Autodesk Inventor part; units mm, degrees
(part 3 of 3)
sketch "Sketch4" plane through (0, 0, 0) normal (0, -1, 0) x (1, 0, 0)
  line L0 (-16.345, -5.1907) -> (6.6347, -5.1907) construction
  line L1 (6.6347, -5.1907) -> (6.6347, -8.929) construction
  line L2 (6.6347, -8.929) -> (-16.345, -8.929) construction
  line L3 (-16.345, -8.929) -> (-16.345, -5.1907) construction
  line L4 (-12.1827, 8.2163) -> (3.5843, 8.2163) construction
  line L5 (3.5843, 8.2163) -> (3.5843, 3.5647) construction
  line L6 (3.5843, 3.5647) -> (-12.1827, 3.5647) construction
  line L7 (-12.1827, 3.5647) -> (-12.1827, 8.2163) construction
  spline S0 degree 2 poles (-8.2562, 3.053) (-8.2439, 2.7183) (-7.9092, 2.4244) (-7.5011, 2.4244) knots 0 0 0 1 2 2 2
  spline S1 degree 2 poles (-7.5011, 2.4244) (-7.3623, 2.4244) (-6.9868, 2.5183) (-6.9133, 2.5551) knots 0 0 0 1 2 2 2
  line L8 (-6.9133, 2.5551) -> (-6.7868, 2.5551)
  line L9 (-6.7868, 2.5551) -> (-6.7868, 1.6734)
  spline S2 degree 2 poles (-6.7868, 1.6734) (-6.9745, 1.6285) (-7.4154, 1.5632) (-7.8684, 1.5632) knots 0 0 0 1 2 2 2
  spline S3 degree 2 poles (-7.8684, 1.5632) (-8.2684, 1.5632) (-8.8602, 1.7632) (-9.0602, 1.9428) knots 0 0 0 1 2 2 2
  spline S4 degree 2 poles (-9.0602, 1.9428) (-9.2521, 2.1224) (-9.448, 2.604) (-9.4643, 2.902) knots 0 0 0 1 2 2 2
  spline S5 degree 2 poles (-9.4643, 2.902) (-10.5827, 2.9673) (-11.8358, 4.3387) (-11.8358, 5.4897) knots 0 0 0 1 2 2 2
  spline S6 degree 2 poles (-11.8358, 5.4897) (-11.8358, 6.6979) (-10.4684, 8.0979) (-9.2602, 8.0979) knots 0 0 0 1 2 2 2
  spline S7 degree 2 poles (-9.2602, 8.0979) (-8.0602, 8.0979) (-6.6847, 6.6979) (-6.6847, 5.4897) knots 0 0 0 1 2 2 2
  spline S8 degree 2 poles (-6.6847, 5.4897) (-6.6847, 4.6) (-7.4888, 3.3102) (-8.2562, 3.053) knots 0 0 0 1 2 2 2
  spline S9 degree 2 poles (-8.3909, 4.2244) (-8.2031, 4.453) (-8.0235, 5.0775) (-8.0235, 5.4938) knots 0 0 0 1 2 2 2
  spline S10 degree 2 poles (-8.0235, 5.4938) (-8.0235, 5.9469) (-8.2317, 6.5755) (-8.399, 6.7714) knots 0 0 0 1 2 2 2
  spline S11 degree 2 poles (-8.399, 6.7714) (-8.5705, 6.9755) (-9.0154, 7.1551) (-9.2602, 7.1551) knots 0 0 0 1 2 2 2
  spline S12 degree 2 poles (-9.2602, 7.1551) (-9.5051, 7.1551) (-9.9378, 6.9795) (-10.1174, 6.7795) knots 0 0 0 1 2 2 2
  spline S13 degree 2 poles (-10.1174, 6.7795) (-10.2847, 6.5918) (-10.497, 5.9306) (-10.497, 5.4938) knots 0 0 0 1 2 2 2
  spline S14 degree 2 poles (-10.497, 5.4938) (-10.497, 5.0448) (-10.2929, 4.4163) (-10.1256, 4.2204) knots 0 0 0 1 2 2 2
  spline S15 degree 2 poles (-10.1256, 4.2204) (-9.9582, 4.0204) (-9.5051, 3.8326) (-9.2602, 3.8326) knots 0 0 0 1 2 2 2
  spline S16 degree 2 poles (-9.2602, 3.8326) (-9.0113, 3.8326) (-8.5623, 4.0244) (-8.3909, 4.2244) knots 0 0 0 1 2 2 2
  line L10 (-2.0113, 2.9918) -> (-3.2235, 2.9918)
  line L11 (-3.2235, 2.9918) -> (-3.2235, 3.4081)
  spline S17 degree 2 poles (-3.2235, 3.4081) (-3.5582, 3.151) (-4.1174, 2.8857) (-4.5011, 2.8857) knots 0 0 0 1 2 2 2
  spline S18 degree 2 poles (-4.5011, 2.8857) (-5.1256, 2.8857) (-5.799, 3.604) (-5.799, 4.3061) knots 0 0 0 1 2 2 2
  line L12 (-5.799, 4.3061) -> (-5.799, 6.7632)
  line L13 (-5.799, 6.7632) -> (-4.5868, 6.7632)
  line L14 (-4.5868, 6.7632) -> (-4.5868, 4.8897)
  spline S19 degree 2 poles (-4.5868, 4.8897) (-4.5868, 4.604) (-4.55, 4.2244) (-4.4807, 4.102) knots 0 0 0 1 2 2 2
  spline S20 degree 2 poles (-4.4807, 4.102) (-4.4194, 3.9755) (-4.1623, 3.8612) (-3.9296, 3.8612) knots 0 0 0 1 2 2 2
  spline S21 degree 2 poles (-3.9296, 3.8612) (-3.7745, 3.8612) (-3.399, 3.9755) (-3.2235, 4.0857) knots 0 0 0 1 2 2 2
  line L15 (-3.2235, 4.0857) -> (-3.2235, 6.7632)
  line L16 (-3.2235, 6.7632) -> (-2.0113, 6.7632)
  line L17 (-2.0113, 6.7632) -> (-2.0113, 2.9918)
  line L18 (0.3438, 2.9918) -> (-0.8684, 2.9918)
  line L19 (-0.8684, 2.9918) -> (-0.8684, 6.7632)
  line L20 (-0.8684, 6.7632) -> (0.3438, 6.7632)
  line L21 (0.3438, 6.7632) -> (0.3438, 2.9918)
  line L22 (0.3765, 7.2979) -> (-0.9011, 7.2979)
  line L23 (-0.9011, 7.2979) -> (-0.9011, 8.2163)
  line L24 (-0.9011, 8.2163) -> (0.3765, 8.2163)
  line L25 (0.3765, 8.2163) -> (0.3765, 7.2979)
  spline S22 degree 2 poles (3.4459, 2.8897) (2.952, 2.8897) (2.1357, 3.1265) (1.8336, 3.3714) knots 0 0 0 1 2 2 2
  spline S23 degree 2 poles (1.8336, 3.3714) (1.5357, 3.6163) (1.2051, 4.3591) (1.2051, 4.8612) knots 0 0 0 1 2 2 2
  spline S24 degree 2 poles (1.2051, 4.8612) (1.2051, 5.3877) (1.5561, 6.1551) (1.8744, 6.404) knots 0 0 0 1 2 2 2
  spline S25 degree 2 poles (1.8744, 6.404) (2.1806, 6.6448) (2.9765, 6.8653) (3.4091, 6.8653) knots 0 0 0 1 2 2 2
  spline S26 degree 2 poles (3.4091, 6.8653) (3.7928, 6.8653) (4.4459, 6.6979) (4.7275, 6.5632) knots 0 0 0 1 2 2 2
  line L26 (4.7275, 6.5632) -> (4.7275, 5.5306)
  line L27 (4.7275, 5.5306) -> (4.5561, 5.5306)
  spline S27 degree 2 poles (4.5561, 5.5306) (4.4867, 5.5918) (4.2867, 5.7551) (4.1438, 5.8326) knots 0 0 0 1 2 2 2
  spline S28 degree 2 poles (4.1438, 5.8326) (4.0051, 5.9061) (3.6785, 6.004) (3.4622, 6.004) knots 0 0 0 1 2 2 2
  spline S29 degree 2 poles (3.4622, 6.004) (2.9765, 6.004) (2.4581, 5.3877) (2.4581, 4.8612) knots 0 0 0 1 2 2 2
  spline S30 degree 2 poles (2.4581, 4.8612) (2.4581, 4.3142) (2.9928, 3.751) (3.4785, 3.751) knots 0 0 0 1 2 2 2
  spline S31 degree 2 poles (3.4785, 3.751) (3.7071, 3.751) (4.0744, 3.8571) (4.1928, 3.9265) knots 0 0 0 1 2 2 2
  spline S32 degree 2 poles (4.1928, 3.9265) (4.3071, 3.9918) (4.4826, 4.1428) (4.5561, 4.2122) knots 0 0 0 1 2 2 2
  line L28 (4.5561, 4.2122) -> (4.7275, 4.2122)
  line L29 (4.7275, 4.2122) -> (4.7275, 3.1836)
  spline S33 degree 2 poles (4.7275, 3.1836) (4.4418, 3.0489) (3.8214, 2.8897) (3.4459, 2.8897) knots 0 0 0 1 2 2 2
  line L30 (9.5275, 2.9918) -> (8.1234, 2.9918)
  line L31 (8.1234, 2.9918) -> (7.0663, 4.6326)
  line L32 (7.0663, 4.6326) -> (6.7398, 4.2285)
  line L33 (6.7398, 4.2285) -> (6.7398, 2.9918)
  line L34 (6.7398, 2.9918) -> (5.5275, 2.9918)
  line L35 (5.5275, 2.9918) -> (5.5275, 8.2163)
  line L36 (5.5275, 8.2163) -> (6.7398, 8.2163)
  line L37 (6.7398, 8.2163) -> (6.7398, 5.1061)
  line L38 (6.7398, 5.1061) -> (8.0336, 6.7632)
  line L39 (8.0336, 6.7632) -> (9.4295, 6.7632)
  line L40 (9.4295, 6.7632) -> (8.0785, 5.1387)
  line L41 (8.0785, 5.1387) -> (9.5275, 2.9918)
  line L42 (12.8744, 5.6122) -> (12.7683, 5.6122)
  spline S34 degree 2 poles (12.7683, 5.6122) (12.6908, 5.6408) (12.3479, 5.6653) (12.2336, 5.6653) knots 0 0 0 1 2 2 2
  spline S35 degree 2 poles (12.2336, 5.6653) (11.9765, 5.6653) (11.5806, 5.6) (11.352, 5.5183) knots 0 0 0 1 2 2 2
  line L43 (11.352, 5.5183) -> (11.352, 2.9918)
  line L44 (11.352, 2.9918) -> (10.1398, 2.9918)
  line L45 (10.1398, 2.9918) -> (10.1398, 6.7632)
  line L46 (10.1398, 6.7632) -> (11.352, 6.7632)
  line L47 (11.352, 6.7632) -> (11.352, 6.2081)
  spline S36 degree 2 poles (11.352, 6.2081) (11.752, 6.551) (12.3398, 6.7755) (12.5887, 6.7755) knots 0 0 0 1 2 2 2
  spline S37 degree 2 poles (12.5887, 6.7755) (12.654, 6.7755) (12.8132, 6.7673) (12.8744, 6.7632) knots 0 0 0 1 2 2 2
  line L48 (12.8744, 6.7632) -> (12.8744, 5.6122)
  line L49 (-13.0732, -8.3254) -> (-14.0161, -8.3254)
  line L50 (-14.0161, -8.3254) -> (-14.834, -7.2258)
  line L51 (-14.834, -7.2258) -> (-15.194, -7.2258)
  line L52 (-15.194, -7.2258) -> (-15.194, -8.3254)
  line L53 (-15.194, -8.3254) -> (-15.963, -8.3254)
  line L54 (-15.963, -8.3254) -> (-15.963, -5.3254)
  line L55 (-15.963, -5.3254) -> (-14.665, -5.3254)
  spline S38 degree 2 poles (-14.665, -5.3254) (-14.3981, -5.3254) (-14.0161, -5.3866) (-13.8495, -5.4871) knots 0 0 0 1 2 2 2
  spline S39 degree 2 poles (-13.8495, -5.4871) (-13.6781, -5.5875) (-13.4797, -5.9083) (-13.4797, -6.1507) knots 0 0 0 1 2 2 2
  spline S40 degree 2 poles (-13.4797, -6.1507) (-13.4797, -6.4813) (-13.7883, -6.9026) (-14.0748, -7.0397) knots 0 0 0 1 2 2 2
  line L56 (-14.0748, -7.0397) -> (-13.0732, -8.3254)
  spline S41 degree 2 poles (-14.2805, -6.2438) (-14.2805, -6.1311) (-14.3736, -5.9695) (-14.4863, -5.923) knots 0 0 0 1 2 2 2
  spline S42 degree 2 poles (-14.4863, -5.923) (-14.5646, -5.8911) (-14.7752, -5.8764) (-14.9148, -5.8764) knots 0 0 0 1 2 2 2
  line L57 (-14.9148, -5.8764) -> (-15.194, -5.8764)
  line L58 (-15.194, -5.8764) -> (-15.194, -6.6846)
  line L59 (-15.194, -6.6846) -> (-14.9565, -6.6846)
  spline S43 degree 2 poles (-14.9565, -6.6846) (-14.7703, -6.6846) (-14.5205, -6.6479) (-14.4348, -6.5842) knots 0 0 0 1 2 2 2
  spline S44 degree 2 poles (-14.4348, -6.5842) (-14.354, -6.5205) (-14.2805, -6.3711) (-14.2805, -6.2438) knots 0 0 0 1 2 2 2
  spline S45 degree 2 poles (-10.4601, -7.194) (-10.4601, -7.7524) (-11.1116, -8.3964) (-11.6993, -8.3964) knots 0 0 0 1 2 2 2
  spline S46 degree 2 poles (-11.6993, -8.3964) (-12.2895, -8.3964) (-12.941, -7.7524) (-12.941, -7.194) knots 0 0 0 1 2 2 2
  spline S47 degree 2 poles (-12.941, -7.194) (-12.941, -6.6332) (-12.2846, -5.9915) (-11.6993, -5.9915) knots 0 0 0 1 2 2 2
  spline S48 degree 2 poles (-11.6993, -5.9915) (-11.1067, -5.9915) (-10.4601, -6.6356) (-10.4601, -7.194) knots 0 0 0 1 2 2 2
  spline S49 degree 2 poles (-11.354, -7.745) (-11.283, -7.6569) (-11.212, -7.4144) (-11.212, -7.1989) knots 0 0 0 1 2 2 2
  spline S50 degree 2 poles (-11.212, -7.1989) (-11.212, -7.0005) (-11.2854, -6.7311) (-11.3491, -6.6503) knots 0 0 0 1 2 2 2
  spline S51 degree 2 poles (-11.3491, -6.6503) (-11.4128, -6.5671) (-11.5965, -6.4985) (-11.6993, -6.4985) knots 0 0 0 1 2 2 2
  spline S52 degree 2 poles (-11.6993, -6.4985) (-11.8046, -6.4985) (-11.9687, -6.5548) (-12.0446, -6.6405) knots 0 0 0 1 2 2 2
  spline S53 degree 2 poles (-12.0446, -6.6405) (-12.1108, -6.7189) (-12.1891, -6.9907) (-12.1891, -7.1989) knots 0 0 0 1 2 2 2
  spline S54 degree 2 poles (-12.1891, -7.1989) (-12.1891, -7.385) (-12.1205, -7.6569) (-12.0544, -7.7377) knots 0 0 0 1 2 2 2
  spline S55 degree 2 poles (-12.0544, -7.7377) (-11.9883, -7.816) (-11.8095, -7.8895) (-11.6944, -7.8895) knots 0 0 0 1 2 2 2
  spline S56 degree 2 poles (-11.6944, -7.8895) (-11.5965, -7.8895) (-11.4152, -7.8234) (-11.354, -7.745) knots 0 0 0 1 2 2 2
  spline S57 degree 2 poles (-7.5801, -7.1622) (-7.5801, -7.696) (-8.1703, -8.3695) (-8.6112, -8.3695) knots 0 0 0 1 2 2 2
  spline S58 degree 2 poles (-8.6112, -8.3695) (-8.7997, -8.3695) (-9.0838, -8.2887) (-9.2136, -8.2128) knots 0 0 0 1 2 2 2
  line L60 (-9.2136, -8.2128) -> (-9.243, -8.3254)
  line L61 (-9.243, -8.3254) -> (-9.941, -8.3254)
  line L62 (-9.941, -8.3254) -> (-9.941, -5.1907)
  line L63 (-9.941, -5.1907) -> (-9.2136, -5.1907)
  line L64 (-9.2136, -5.1907) -> (-9.2136, -6.3001)
  spline S59 degree 2 poles (-9.2136, -6.3001) (-9.0471, -6.1654) (-8.6993, -6.0013) (-8.4716, -6.0013) knots 0 0 0 1 2 2 2
  spline S60 degree 2 poles (-8.4716, -6.0013) (-8.043, -6.0013) (-7.5801, -6.6185) (-7.5801, -7.1622) knots 0 0 0 1 2 2 2
  spline S61 degree 2 poles (-8.3271, -7.1793) (-8.3271, -6.8781) (-8.5328, -6.5524) (-8.7948, -6.5524) knots 0 0 0 1 2 2 2
  spline S62 degree 2 poles (-8.7948, -6.5524) (-8.8977, -6.5524) (-9.1157, -6.6136) (-9.2136, -6.6724) knots 0 0 0 1 2 2 2
  line L65 (-9.2136, -6.6724) -> (-9.2136, -7.8038)
  spline S63 degree 2 poles (-9.2136, -7.8038) (-9.1352, -7.8332) (-8.9957, -7.8528) (-8.8952, -7.8528) knots 0 0 0 1 2 2 2
  spline S64 degree 2 poles (-8.8952, -7.8528) (-8.6087, -7.8528) (-8.3271, -7.5148) (-8.3271, -7.1793) knots 0 0 0 1 2 2 2
  spline S65 degree 2 poles (-4.7418, -7.194) (-4.7418, -7.7524) (-5.3932, -8.3964) (-5.981, -8.3964) knots 0 0 0 1 2 2 2
  spline S66 degree 2 poles (-5.981, -8.3964) (-6.5712, -8.3964) (-7.2226, -7.7524) (-7.2226, -7.194) knots 0 0 0 1 2 2 2
  spline S67 degree 2 poles (-7.2226, -7.194) (-7.2226, -6.6332) (-6.5663, -5.9915) (-5.981, -5.9915) knots 0 0 0 1 2 2 2
  spline S68 degree 2 poles (-5.981, -5.9915) (-5.3883, -5.9915) (-4.7418, -6.6356) (-4.7418, -7.194) knots 0 0 0 1 2 2 2
  spline S69 degree 2 poles (-5.6357, -7.745) (-5.5646, -7.6569) (-5.4936, -7.4144) (-5.4936, -7.1989) knots 0 0 0 1 2 2 2
  spline S70 degree 2 poles (-5.4936, -7.1989) (-5.4936, -7.0005) (-5.5671, -6.7311) (-5.6308, -6.6503) knots 0 0 0 1 2 2 2
  spline S71 degree 2 poles (-5.6308, -6.6503) (-5.6944, -6.5671) (-5.8781, -6.4985) (-5.981, -6.4985) knots 0 0 0 1 2 2 2
  spline S72 degree 2 poles (-5.981, -6.4985) (-6.0863, -6.4985) (-6.2503, -6.5548) (-6.3263, -6.6405) knots 0 0 0 1 2 2 2
  spline S73 degree 2 poles (-6.3263, -6.6405) (-6.3924, -6.7189) (-6.4708, -6.9907) (-6.4708, -7.1989) knots 0 0 0 1 2 2 2
  spline S74 degree 2 poles (-6.4708, -7.1989) (-6.4708, -7.385) (-6.4022, -7.6569) (-6.3361, -7.7377) knots 0 0 0 1 2 2 2
  spline S75 degree 2 poles (-6.3361, -7.7377) (-6.2699, -7.816) (-6.0912, -7.8895) (-5.9761, -7.8895) knots 0 0 0 1 2 2 2
  spline S76 degree 2 poles (-5.9761, -7.8895) (-5.8781, -7.8895) (-5.6969, -7.8234) (-5.6357, -7.745) knots 0 0 0 1 2 2 2
  spline S77 degree 2 poles (-1.6144, -7.4071) (-1.6144, -7.625) (-1.7908, -7.9679) (-1.9426, -8.0805) knots 0 0 0 1 2 2 2
  spline S78 degree 2 poles (-1.9426, -8.0805) (-2.1214, -8.2128) (-2.545, -8.3254) (-2.8732, -8.3254) knots 0 0 0 1 2 2 2
  line L66 (-2.8732, -8.3254) -> (-4.1834, -8.3254)
  line L67 (-4.1834, -8.3254) -> (-4.1834, -5.3254)
  line L68 (-4.1834, -5.3254) -> (-3.0177, -5.3254)
  spline S79 degree 2 poles (-3.0177, -5.3254) (-2.6552, -5.3254) (-2.3197, -5.3744) (-2.1532, -5.4552) knots 0 0 0 1 2 2 2
  spline S80 degree 2 poles (-2.1532, -5.4552) (-1.9818, -5.5434) (-1.8152, -5.8348) (-1.8152, -6.0234) knots 0 0 0 1 2 2 2
  spline S81 degree 2 poles (-1.8152, -6.0234) (-1.8152, -6.2413) (-2.0454, -6.572) (-2.2561, -6.665) knots 0 0 0 1 2 2 2
  line L69 (-2.2561, -6.665) -> (-2.2561, -6.6822)
  spline S82 degree 2 poles (-2.2561, -6.6822) (-1.9597, -6.7409) (-1.6144, -7.1058) (-1.6144, -7.4071) knots 0 0 0 1 2 2 2
  spline S83 degree 2 poles (-2.4177, -7.3948) (-2.4177, -7.2503) (-2.5279, -7.096) (-2.6626, -7.0569) knots 0 0 0 1 2 2 2
  spline S84 degree 2 poles (-2.6626, -7.0569) (-2.7532, -7.0324) (-3.0716, -7.0275) (-3.2454, -7.0275) knots 0 0 0 1 2 2 2
  line L70 (-3.2454, -7.0275) -> (-3.4144, -7.0275)
  line L71 (-3.4144, -7.0275) -> (-3.4144, -7.7744)
  line L72 (-3.4144, -7.7744) -> (-3.3581, -7.7744)
  spline S85 degree 2 poles (-3.3581, -7.7744) (-3.0299, -7.7744) (-2.7483, -7.7695) (-2.6308, -7.7205) knots 0 0 0 1 2 2 2
  spline S86 degree 2 poles (-2.6308, -7.7205) (-2.5083, -7.6691) (-2.4177, -7.5026) (-2.4177, -7.3948) knots 0 0 0 1 2 2 2
  spline S87 degree 2 poles (-2.6063, -6.1752) (-2.6063, -6.0993) (-2.6822, -5.9499) (-2.7752, -5.9156) knots 0 0 0 1 2 2 2
  spline S88 degree 2 poles (-2.7752, -5.9156) (-2.861, -5.8813) (-3.1132, -5.8764) (-3.341, -5.8764) knots 0 0 0 1 2 2 2
  line L73 (-3.341, -5.8764) -> (-3.4144, -5.8764)
  line L74 (-3.4144, -5.8764) -> (-3.4144, -6.5107)
  line L75 (-3.4144, -6.5107) -> (-3.292, -6.5107)
  spline S89 degree 2 poles (-3.292, -6.5107) (-3.1083, -6.5107) (-2.8512, -6.4985) (-2.7752, -6.4642) knots 0 0 0 1 2 2 2
  spline S90 degree 2 poles (-2.7752, -6.4642) (-2.6699, -6.4177) (-2.6063, -6.2707) (-2.6063, -6.1752) knots 0 0 0 1 2 2 2
  line L76 (0.5627, -6.7532) -> (0.499, -6.7532)
  spline S91 degree 2 poles (0.499, -6.7532) (0.4525, -6.736) (0.2468, -6.7213) (0.1782, -6.7213) knots 0 0 0 1 2 2 2
  spline S92 degree 2 poles (0.1782, -6.7213) (0.0239, -6.7213) (-0.2136, -6.7605) (-0.3508, -6.8095) knots 0 0 0 1 2 2 2
  line L77 (-0.3508, -6.8095) -> (-0.3508, -8.3254)
  line L78 (-0.3508, -8.3254) -> (-1.0781, -8.3254)
  line L79 (-1.0781, -8.3254) -> (-1.0781, -6.0626)
  line L80 (-1.0781, -6.0626) -> (-0.3508, -6.0626)
  line L81 (-0.3508, -6.0626) -> (-0.3508, -6.3956)
  spline S93 degree 2 poles (-0.3508, -6.3956) (-0.1108, -6.1899) (0.2419, -6.0552) (0.3913, -6.0552) knots 0 0 0 1 2 2 2
  spline S94 degree 2 poles (0.3913, -6.0552) (0.4305, -6.0552) (0.526, -6.0601) (0.5627, -6.0626) knots 0 0 0 1 2 2 2
  line L82 (0.5627, -6.0626) -> (0.5627, -6.7532)
  line L83 (2.615, -6.7532) -> (2.5513, -6.7532)
  spline S95 degree 2 poles (2.5513, -6.7532) (2.5048, -6.736) (2.299, -6.7213) (2.2305, -6.7213) knots 0 0 0 1 2 2 2
  spline S96 degree 2 poles (2.2305, -6.7213) (2.0762, -6.7213) (1.8386, -6.7605) (1.7015, -6.8095) knots 0 0 0 1 2 2 2
  line L84 (1.7015, -6.8095) -> (1.7015, -8.3254)
  line L85 (1.7015, -8.3254) -> (0.9741, -8.3254)
  line L86 (0.9741, -8.3254) -> (0.9741, -6.0626)
  line L87 (0.9741, -6.0626) -> (1.7015, -6.0626)
  line L88 (1.7015, -6.0626) -> (1.7015, -6.3956)
  spline S97 degree 2 poles (1.7015, -6.3956) (1.9415, -6.1899) (2.2941, -6.0552) (2.4435, -6.0552) knots 0 0 0 1 2 2 2
  spline S98 degree 2 poles (2.4435, -6.0552) (2.4827, -6.0552) (2.5782, -6.0601) (2.615, -6.0626) knots 0 0 0 1 2 2 2
  line L89 (2.615, -6.0626) -> (2.615, -6.7532)
  line L90 (5.2256, -8.3254) -> (4.4982, -8.3254)
  line L91 (4.4982, -8.3254) -> (4.4982, -8.0903)
  spline S99 degree 2 poles (4.4982, -8.0903) (4.3121, -8.2422) (3.9864, -8.3891) (3.7709, -8.3891) knots 0 0 0 1 2 2 2
  spline S100 degree 2 poles (3.7709, -8.3891) (3.3595, -8.3891) (2.8648, -7.7524) (2.8648, -7.2111) knots 0 0 0 1 2 2 2
  spline S101 degree 2 poles (2.8648, -7.2111) (2.8648, -6.9246) (3.0313, -6.4789) (3.1758, -6.3197) knots 0 0 0 1 2 2 2
  spline S102 degree 2 poles (3.1758, -6.3197) (3.3129, -6.1679) (3.7048, -6.0013) (3.8982, -6.0013) knots 0 0 0 1 2 2 2
  spline S103 degree 2 poles (3.8982, -6.0013) (4.1015, -6.0013) (4.3611, -6.0871) (4.4982, -6.1556) knots 0 0 0 1 2 2 2
  line L92 (4.4982, -6.1556) -> (4.4982, -5.1907)
  line L93 (4.4982, -5.1907) -> (5.2256, -5.1907)
  line L94 (5.2256, -5.1907) -> (5.2256, -8.3254)
  line L95 (4.4982, -7.7034) -> (4.4982, -6.5915)
  spline S104 degree 2 poles (4.4982, -6.5915) (4.4223, -6.5597) (4.2533, -6.5303) (4.1823, -6.5303) knots 0 0 0 1 2 2 2
  spline S105 degree 2 poles (4.1823, -6.5303) (3.8982, -6.5303) (3.6117, -6.8879) (3.6117, -7.2038) knots 0 0 0 1 2 2 2
  spline S106 degree 2 poles (3.6117, -7.2038) (3.6117, -7.5369) (3.8419, -7.8381) (4.0941, -7.8381) knots 0 0 0 1 2 2 2
  spline S107 degree 2 poles (4.0941, -7.8381) (4.1921, -7.8381) (4.415, -7.7646) (4.4982, -7.7034) knots 0 0 0 1 2 2 2
  line L96 (6.6925, -8.3254) -> (5.9382, -8.3254)
  line L97 (5.9382, -8.3254) -> (5.9382, -7.5344)
  line L98 (5.9382, -7.5344) -> (6.6925, -7.5344)
  line L99 (6.6925, -7.5344) -> (6.6925, -8.3254)
  spline S108 degree 2 poles (8.5807, -8.3866) (8.2843, -8.3866) (7.7946, -8.2446) (7.6133, -8.0977) knots 0 0 0 1 2 2 2
  spline S109 degree 2 poles (7.6133, -8.0977) (7.4346, -7.9507) (7.2362, -7.505) (7.2362, -7.2038) knots 0 0 0 1 2 2 2
  spline S110 degree 2 poles (7.2362, -7.2038) (7.2362, -6.8879) (7.4468, -6.4275) (7.6378, -6.2781) knots 0 0 0 1 2 2 2
  spline S111 degree 2 poles (7.6378, -6.2781) (7.8215, -6.1336) (8.299, -6.0013) (8.5586, -6.0013) knots 0 0 0 1 2 2 2
  spline S112 degree 2 poles (8.5586, -6.0013) (8.7888, -6.0013) (9.1807, -6.1017) (9.3497, -6.1826) knots 0 0 0 1 2 2 2
  line L100 (9.3497, -6.1826) -> (9.3497, -6.8022)
  line L101 (9.3497, -6.8022) -> (9.2468, -6.8022)
  spline S113 degree 2 poles (9.2468, -6.8022) (9.2052, -6.7654) (9.0852, -6.6675) (8.9995, -6.6209) knots 0 0 0 1 2 2 2
  spline S114 degree 2 poles (8.9995, -6.6209) (8.9162, -6.5768) (8.7203, -6.5181) (8.5905, -6.5181) knots 0 0 0 1 2 2 2
  spline S115 degree 2 poles (8.5905, -6.5181) (8.299, -6.5181) (7.988, -6.8879) (7.988, -7.2038) knots 0 0 0 1 2 2 2
  spline S116 degree 2 poles (7.988, -7.2038) (7.988, -7.532) (8.3088, -7.8699) (8.6003, -7.8699) knots 0 0 0 1 2 2 2
  spline S117 degree 2 poles (8.6003, -7.8699) (8.7374, -7.8699) (8.9578, -7.8062) (9.0288, -7.7646) knots 0 0 0 1 2 2 2
  spline S118 degree 2 poles (9.0288, -7.7646) (9.0974, -7.7254) (9.2027, -7.6348) (9.2468, -7.5932) knots 0 0 0 1 2 2 2
  line L102 (9.2468, -7.5932) -> (9.3497, -7.5932)
  line L103 (9.3497, -7.5932) -> (9.3497, -8.2103)
  spline S119 degree 2 poles (9.3497, -8.2103) (9.1782, -8.2911) (8.806, -8.3866) (8.5807, -8.3866) knots 0 0 0 1 2 2 2
  spline S120 degree 2 poles (12.1439, -7.194) (12.1439, -7.7524) (11.4925, -8.3964) (10.9048, -8.3964) knots 0 0 0 1 2 2 2
  spline S121 degree 2 poles (10.9048, -8.3964) (10.3146, -8.3964) (9.6631, -7.7524) (9.6631, -7.194) knots 0 0 0 1 2 2 2
  spline S122 degree 2 poles (9.6631, -7.194) (9.6631, -6.6332) (10.3195, -5.9915) (10.9048, -5.9915) knots 0 0 0 1 2 2 2
  spline S123 degree 2 poles (10.9048, -5.9915) (11.4974, -5.9915) (12.1439, -6.6356) (12.1439, -7.194) knots 0 0 0 1 2 2 2
  spline S124 degree 2 poles (11.2501, -7.745) (11.3211, -7.6569) (11.3921, -7.4144) (11.3921, -7.1989) knots 0 0 0 1 2 2 2
  spline S125 degree 2 poles (11.3921, -7.1989) (11.3921, -7.0005) (11.3186, -6.7311) (11.255, -6.6503) knots 0 0 0 1 2 2 2
  spline S126 degree 2 poles (11.255, -6.6503) (11.1913, -6.5671) (11.0076, -6.4985) (10.9048, -6.4985) knots 0 0 0 1 2 2 2
  spline S127 degree 2 poles (10.9048, -6.4985) (10.7995, -6.4985) (10.6354, -6.5548) (10.5595, -6.6405) knots 0 0 0 1 2 2 2
  spline S128 degree 2 poles (10.5595, -6.6405) (10.4933, -6.7189) (10.415, -6.9907) (10.415, -7.1989) knots 0 0 0 1 2 2 2
  spline S129 degree 2 poles (10.415, -7.1989) (10.415, -7.385) (10.4835, -7.6569) (10.5497, -7.7377) knots 0 0 0 1 2 2 2
  spline S130 degree 2 poles (10.5497, -7.7377) (10.6158, -7.816) (10.7946, -7.8895) (10.9097, -7.8895) knots 0 0 0 1 2 2 2
  spline S131 degree 2 poles (10.9097, -7.8895) (11.0076, -7.8895) (11.1888, -7.8234) (11.2501, -7.745) knots 0 0 0 1 2 2 2
  line L104 (14.8721, -6.7213) -> (14.8721, -8.3254)
  line L105 (14.8721, -8.3254) -> (14.1448, -8.3254)
  line L106 (14.1448, -8.3254) -> (14.1448, -7.194)
  spline S132 degree 2 poles (14.1448, -7.194) (14.1448, -7.0299) (14.1276, -6.7973) (14.0933, -6.7262) knots 0 0 0 1 2 2 2
  spline S133 degree 2 poles (14.0933, -6.7262) (14.0566, -6.6528) (13.9097, -6.5866) (13.7774, -6.5866) knots 0 0 0 1 2 2 2
  spline S134 degree 2 poles (13.7774, -6.5866) (13.6697, -6.5866) (13.4688, -6.6724) (13.388, -6.7213) knots 0 0 0 1 2 2 2
  line L107 (13.388, -6.7213) -> (13.388, -8.3254)
  line L108 (13.388, -8.3254) -> (12.6607, -8.3254)
  line L109 (12.6607, -8.3254) -> (12.6607, -6.0626)
  line L110 (12.6607, -6.0626) -> (13.388, -6.0626)
  line L111 (13.388, -6.0626) -> (13.388, -6.3124)
  spline S135 degree 2 poles (13.388, -6.3124) (13.5741, -6.1654) (13.917, -6.0013) (14.1252, -6.0013) knots 0 0 0 1 2 2 2
  spline S136 degree 2 poles (14.1252, -6.0013) (14.348, -6.0013) (14.6884, -6.1997) (14.7864, -6.3932) knots 0 0 0 1 2 2 2
  spline S137 degree 2 poles (14.7864, -6.3932) (15.0019, -6.212) (15.4133, -6.0013) (15.6092, -6.0013) knots 0 0 0 1 2 2 2
  spline S138 degree 2 poles (15.6092, -6.0013) (15.9766, -6.0013) (16.3562, -6.4397) (16.3562, -6.8536) knots 0 0 0 1 2 2 2
  line L112 (16.3562, -6.8536) -> (16.3562, -8.3254)
  line L113 (16.3562, -8.3254) -> (15.6288, -8.3254)
  line L114 (15.6288, -8.3254) -> (15.6288, -7.194)
  spline S139 degree 2 poles (15.6288, -7.194) (15.6288, -7.0275) (15.6141, -6.7973) (15.5774, -6.7262) knots 0 0 0 1 2 2 2
  spline S140 degree 2 poles (15.5774, -6.7262) (15.5431, -6.6528) (15.3962, -6.5866) (15.2615, -6.5866) knots 0 0 0 1 2 2 2
  spline S141 degree 2 poles (15.2615, -6.5866) (15.1709, -6.5866) (14.997, -6.6479) (14.8721, -6.7213) knots 0 0 0 1 2 2 2
  point P0 (0, 0)
  constraints: 4 other
emboss "Emboss1" sketch "Sketch4" operation cut depth 0.54 direction (0, 1, 0)
body "Solid1"
